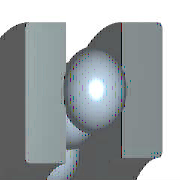
# Autodesk Inventor part: ISO 104 - 1 71 - 10 x 24 x 6
Saved by Autodesk Inventor 2023.3 (Build 273359000, 359)
## iProperties
Created: 2022-02-04
Part Number: ISO 104 - 1 71 - 10 x 24 x 6
Material: Steel, Mild
Description: Rolling bearing-Thrust bearing(Single Direction)
Document SubType Name: Modeling
Standard: ISO 104
Designer: Csábi-Kis Henrik
Standard Revision: Third edition 2002-02-01
Standards Organization: ISO
Language: en-US
Size Designation: 1 71 - 10 x 24 x 6
Categories: <MemberInstance><Categories><Category DisplayName="Shaft Parts" InternalName="7f7aeb1f-a693-4053-b835-cee3144e0d98" Mnemonic="SHFT"><Category DisplayName="Bearings" InternalName="242d30a3-7172-44e6-a363-b0a3d8f1b556" Mnemonic="BRNG"><CategoryParameter DisplayName="Width" InternalName="25fc5f6e-338b-4801-b5ed-8959743e396e" Mnemonic="wdth"/><CategoryParameter DisplayName="Size Designation" InternalName="2c4e891a-c8f4-49ed-a5c1-5131476c6feb" Mnemonic="sizedes"/><CategoryParameter DisplayName="Basic Dynamic Load Rating" InternalName="440972dd-7009-4861-bd45-69ffbb461423" Mnemonic="bdynlrat"/><CategoryParameter DisplayName="Shaft Diameter" InternalName="91302473-2833-4451-a660-c5d4a8d6a031" Mnemonic="shaftdia"/><CategoryParameter DisplayName="Touch Angle" InternalName="aa21a452-7974-4a55-b5cf-1c2972de2aea" Mnemonic="TouchAngle"/><CategoryParameter DisplayName="Outer Diameter" InternalName="d441686c-04bd-4681-b674-94fbc173ec23" Mnemonic="outdia"/><Category DisplayName="Ball Bearings" InternalName="9b553946-0899-4a5e-a403-c1d9295e77c1" Mnemonic="BALLBEAR"><CategoryParameter DisplayName="Radial Dynamic Load Factor when Fa/Fr &lt;= e" InternalName="051e59b3-bd55-4dad-8b07-38b5cb912881" Mnemonic="raddynfc1"/><CategoryParameter DisplayName="Basic Static Load Rating" InternalName="0f13fbbf-c511-4d43-b4c7-197b47424baf" Mnemonic="bstatlrat"/><CategoryParameter DisplayName="Exponent for Determining Life" InternalName="3029e2ef-9460-4be8-bdfd-dfe61437473d" Mnemonic="lifeexp"/><CategoryParameter DisplayName="Friction Factor" InternalName="3086b0f2-3d69-46ff-8a75-fe12e395bb47" Mnemonic="fricfct"/><CategoryParameter DisplayName="Min. Shaft Diameter" InternalName="4a5be9bc-ad86-4bf2-8167-102dad5d3e27" Mnemonic="minshaftdia"/><CategoryParameter DisplayName="Axial Dynamic Load Factor when Fa/Fr &gt; e" InternalName="4b6ff741-5956-4a40-80f5-34eb9259f88c" Mnemonic="axdynfc2"/><CategoryParameter DisplayName="Limiting Speed Lubrication Grease" InternalName="5237843b-2c8d-46d3-8227-f3e9dd85a12e" Mnemonic="lubgrsp"/><CategoryParameter DisplayName="Limiting Speed Oil" InternalName="60628548-8907-44dc-8e09-603d72f5766f" Mnemonic="oilspd"/><CategoryParameter DisplayName="Axial Static Load Factor" InternalName="74dbf5e2-8362-409a-802f-3c2235668d99" Mnemonic="axdynfc0"/><CategoryParameter DisplayName="Mass" InternalName="7b80f85c-da81-4dea-b8db-d7c689da91b2" Mnemonic="mass"/><CategoryParameter DisplayName="Radius" InternalName="83352640-dfae-4cba-bc9f-11ecbfb0001c" Mnemonic="rad"/><CategoryParameter DisplayName="Radial Static Load Factor" InternalName="83ce084d-c51e-4598-a871-e8e1e34b26ee" Mnemonic="raddynfc0"/><CategoryParameter DisplayName="Axial Dynamic Load Factor when Fa/Fr &lt;= e" InternalName="ae45a7db-08df-4411-99a8-2f035015bff9" Mnemonic="axdynfc1"/><CategoryParameter DisplayName="Max. Hub Step Diameter" InternalName="b5cf89e0-ca87-439c-b08c-a25e2999ab06" Mnemonic="maxhubdia"/><CategoryParameter DisplayName="Limiting Value for Factor Determination" InternalName="be0ce6fc-cad4-4218-b484-c34dd2571812" Mnemonic="limvalfac"/><CategoryParameter DisplayName="Radial Dynamic Load Factor when Fa/Fr &gt; e" InternalName="e513bdb7-139f-4b3c-af32-49e0ba1226b9" Mnemonic="raddynfc2"/><CategoryParameter DisplayName="Max. Step Fillet Radius" InternalName="f6ce6695-cf2c-4ec9-8d20-66671e0e35a4" Mnemonic="maxstprad"/><Category DisplayName="Thrust Ball Bearings" InternalName="fd9b3ea9-37cc-4212-9aeb-e74e3b8fad91" Mnemonic="BBTBB"/></Category></Category></Category><Category DisplayName="DataType" InternalName="23b78d0f-2648-40c6-8793-ca6db495c9e8" Mnemonic="DATATYPE"><CategoryParameter DisplayName="DisplayName" InternalName="05415f3d-3907-474b-a020-eb9d644f4cf3" Mnemonic="DISPLAYNAME"/><CategoryParameter DisplayName="Standard" InternalName="0c0a119c-1e12-4c84-803f-101930972f5e" Mnemonic="STANDARD"/><CategoryParameter DisplayName="Description" InternalName="13903e3d-64b1-4950-80da-f627842ea37f" Mnemonic="DESCRIPTION"/><CategoryParameter DisplayName="Designation" InternalName="2675968c-4ce5-49e0-a4f5-552d29089031" Mnemonic="DESIGNATION"/><CategoryParameter DisplayName="Default Row" InternalName="2af9ec52-faaa-4026-b378-f9fa4afca842" Mnemonic="DEFAULTROW"/><CategoryParameter DisplayName="Folder Name" InternalName="3f06958e-8713-4116-9be7-ed6184ecc97b" Mnemonic="FOLDERNAME"/><CategoryParameter DisplayName="Revision Guid" InternalName="45a75005-10b1-4dfc-8d6d-dfe629f0b93c" Mnemonic="REVISIONGUID"/><CategoryParameter DisplayName="FileName" InternalName="8b46a4cc-9585-4fed-90c3-899f57e09a73" Mnemonic="FILENAME"/><CategoryParameter DisplayName="StdsOrg" InternalName="8f5914e1-4693-403f-8ab5-d37768198c9d" Mnemonic="STDSORG"/><CategoryParameter DisplayName="Family Version" InternalName="914462f6-6e19-4b14-ba84-155b9680b1d0" Mnemonic="FAMILYREVISION"/><CategoryParameter DisplayName="Standard Revision" InternalName="91d5a463-65c2-4fde-b823-3b7fea5e8e17" Mnemonic="STANDARDREVISION"/><CategoryParameter DisplayName="Member Revision" InternalName="a65d44b9-392f-4f4f-857b-e4b3d54996fe" Mnemonic="MEMBERREVISION"/><CategoryParameter DisplayName="ClipFormat" InternalName="bc51e27b-3422-4e78-93ef-cec197ddf230" Mnemonic="CLIPFORMAT"/><CategoryParameter DisplayName="Manufacturer" InternalName="cd6c7a72-a28a-4e50-99a9-2c7f4e13e5ad" Mnemonic="MANUFACTURER"/><CategoryParameter DisplayName="InternalName" InternalName="cf1d0246-76d9-4b4a-8305-fa0409afb5c1" Mnemonic="INTERNALNAME"/><CategoryParameter DisplayName="IsMetric" InternalName="e2385c5b-1ea4-4823-96a8-8de651266ec3" Mnemonic="ISMETRIC"/><Category DisplayName="Part" InternalName="c0e0b642-3bcb-4cc8-9e80-f96d35c4afa4" Mnemonic="PART"><CategoryParameter DisplayName="Part Number" InternalName="016b6077-bfbe-49bd-92c9-d8d59c39c941" Mnemonic="PARTNUMBER"/><CategoryParameter DisplayName="Stock Number" InternalName="4dba7c1c-e26c-444e-836c-b08b433409a8" Mnemonic="STOCKNUMBER"/><CategoryParameter DisplayName="Material Key" InternalName="5c9a8adb-dd2b-4535-b97f-0a94a95fe41f" Mnemonic="MATERIALKEY"/><CategoryParameter DisplayName="Material" InternalName="818a152a-d3c3-49ca-80ee-df7d91421b8e" Mnemonic="MATERIAL"/></Category></Category><Category DisplayName="LegacyMap" InternalName="cd87c42b-3e48-431e-b5c0-1cbeb14dfe77" Mnemonic="LEGACYMAP"><CategoryParameter DisplayName="unique DA member ID" InternalName="0918ad47-427f-4fed-ae26-24c81c58f590" Mnemonic="DACOOKIE"/><CategoryParameter DisplayName="Merge11 ID" InternalName="0ee8fb18-e2ed-4f39-96f6-1f4b5f50aa71" Mnemonic="MERGE11"/><CategoryParameter DisplayName="unique CC member ID" InternalName="5193edd4-b2b0-4ab4-9d54-de900eee34e0" Mnemonic="CCCOOKIE"/><CategoryParameter DisplayName="Split ID" InternalName="72b5c83c-be7f-45c4-ae51-9160ea6deb26" Mnemonic="SPLIT"/><CategoryParameter DisplayName="MemberID" InternalName="8e5e0294-fc51-4c8f-b3d7-003dc5ed94f6" Mnemonic="MEMBERID"/><CategoryParameter DisplayName="CatalogName" InternalName="d99d1e27-aa94-4de2-af4c-c348882a6f4f" Mnemonic="CATALOGNAME"/><CategoryParameter DisplayName="FamilyNumber" InternalName="e705e1f4-09cb-413e-91f9-551b4188271e" Mnemonic="FAMILYNUMBER"/></Category></Categories><FamilyTemplate Id="ba0018"><FamilyTemplateParameters><FamilyTemplateParameter ObjectType="kUserParameterObject" ValueType="xs:double" Id="1" ObjectReferenceKey="WR"/><FamilyTemplateParameter ObjectType="kUserParameterObject" ValueType="xs:double" Id="2" ObjectReferenceKey="BC"/><FamilyTemplateParameter ObjectType="kUserParameterObject" ValueType="xs:double" Id="3" ObjectReferenceKey="KRS"/><FamilyTemplateParameter ObjectType="kUserParameterObject" ValueType="xs:double" Id="4" ObjectReferenceKey="WD"/><FamilyTemplateParameter ObjectType="kUserParameterObject" ValueType="xs:double" Id="5" ObjectReferenceKey="KAD1"/><FamilyTemplateParameter ObjectType="kUserParameterObject" ValueType="xs:double" Id="6" ObjectReferenceKey="KB"/><FamilyTemplateParameter ObjectType="kUserParameterObject" ValueType="xs:double" Id="7" ObjectReferenceKey="BBA"/><FamilyTemplateParameter ObjectType="kUserParameterObject" ValueType="xs:double" Id="8" ObjectReferenceKey="BC0"/><FamilyTemplateParameter ObjectType="kUserParameterObject" ValueType="xs:double" Id="9" ObjectReferenceKey="BD"/><FamilyTemplateParameter ObjectType="kUserParameterObject" ValueType="xs:double" Id="10" ObjectReferenceKey="BR"/><FamilyTemplateParameter ObjectType="kUserParameterObject" ValueType="xs:double" Id="11" ObjectReferenceKey="KID1"/><FamilyTemplateParameter ObjectType="kUserParameterObject" ValueType="xs:double" Id="12" ObjectReferenceKey="BI"/><FamilyTemplateParameter ObjectType="kPropertyObject" ValueType="xs:string" Id="100" ObjectReferenceKey="{32853F0F-3444-11d1-9E93-0060B03C1CA6}" SubObjectId="52"/><FamilyTemplateParameter ObjectType="kPropertyObject" ValueType="xs:string" Id="105" ObjectReferenceKey="{32853F0F-3444-11d1-9E93-0060B03C1CA6}" SubObjectId="5"/><FamilyTemplateParameter ObjectType="kPartComponentDefinitionObject" ValueType="xs:string" Id="110" SubObjectId="Material"/></FamilyTemplateParameters></FamilyTemplate><CategoryParameterMap><ParamToTemplateMap><ParamToTemplate CategoryParameter="//CategoryParameter[@InternalName='05415f3d-3907-474b-a020-eb9d644f4cf3']" ConstantValue="ISO 104 (Single Direction)"/><ParamToTemplate CategoryParameter="//CategoryParameter[@InternalName='cf1d0246-76d9-4b4a-8305-fa0409afb5c1']" ConstantValue="14b0c8a4-116f-4d89-bad3-372984a9f60c"/><ParamToTemplate CategoryParameter="//CategoryParameter[@InternalName='3f06958e-8713-4116-9be7-ed6184ecc97b']" ConstantValue="ISO 104"/><ParamToTemplate CategoryParameter="//CategoryParameter[@InternalName='914462f6-6e19-4b14-ba84-155b9680b1d0']" ConstantValue="10"/><ParamToTemplate CategoryParameter="//CategoryParameter[@InternalName='bc51e27b-3422-4e78-93ef-cec197ddf230']" ConstantValue="CF_INVENTOR.STDPARTS"/><ParamToTemplate CategoryParameter="//CategoryParameter[@InternalName='e2385c5b-1ea4-4823-96a8-8de651266ec3']" ConstantValue="true"/><ParamToTemplate CategoryParameter="//CategoryParameter[@InternalName='13903e3d-64b1-4950-80da-f627842ea37f']" ConstantValue="Rolling bearing-Thrust bearing(Single Direction)"/><ParamToTemplate CategoryParameter="//CategoryParameter[@InternalName='8f5914e1-4693-403f-8ab5-d37768198c9d']" ConstantValue="ISO"/><ParamToTemplate CategoryParameter="//CategoryParameter[@InternalName='0c0a119c-1e12-4c84-803f-101930972f5e']" ConstantValue="ISO 104"/><ParamToTemplate CategoryParameter="//CategoryParameter[@InternalName='cd6c7a72-a28a-4e50-99a9-2c7f4e13e5ad']" TemplateParameter="104"/><ParamToTemplate CategoryParameter="//CategoryParameter[@InternalName='91d5a463-65c2-4fde-b823-3b7fea5e8e17']" ConstantValue="Third edition 2002-02-01"/><ParamToTemplate CategoryParameter="//CategoryParameter[@InternalName='45a75005-10b1-4dfc-8d6d-dfe629f0b93c']" ConstantValue="254451d5-769d-4a13-b570-04789f9de70c"/><ParamToTemplate CategoryParameter="//CategoryParameter[@InternalName='2af9ec52-faaa-4026-b378-f9fa4afca842']" ConstantValue="10"/><ParamToTemplate CategoryParameter="//CategoryParameter[@InternalName='d99d1e27-aa94-4de2-af4c-c348882a6f4f']" ConstantValue="ISO"/><ParamToTemplate CategoryParameter="//CategoryParameter[@InternalName='e705e1f4-09cb-413e-91f9-551b4188271e']" ConstantValue="112"/><ParamToTemplate CategoryParameter="//CategoryParameter[@InternalName='8b46a4cc-9585-4fed-90c3-899f57e09a73']" ConstantValue="ISO 104 - 1 71 - 10 x 24 x 6"/><ParamToTemplate CategoryParameter="//CategoryParameter[@InternalName='a65d44b9-392f-4f4f-857b-e4b3d54996fe']" ConstantValue="9b549998-5bd1-48f5-9ed4-53cb02577c6e"/><ParamToTemplate CategoryParameter="//CategoryParameter[@InternalName='2c4e891a-c8f4-49ed-a5c1-5131476c6feb']" ConstantValue="1 71 - 10 x 24 x 6"/><ParamToTemplate CategoryParameter="//CategoryParameter[@InternalName='8e5e0294-fc51-4c8f-b3d7-003dc5ed94f6']" ConstantValue="210"/><ParamToTemplate CategoryParameter="//CategoryParameter[@InternalName='aa21a452-7974-4a55-b5cf-1c2972de2aea']" TemplateParameter="7"/><ParamToTemplate CategoryParameter="//CategoryParameter[@InternalName='440972dd-7009-4861-bd45-69ffbb461423']" TemplateParameter="2"/><ParamToTemplate CategoryParameter="//CategoryParameter[@InternalName='0f13fbbf-c511-4d43-b4c7-197b47424baf']" TemplateParameter="8"/><ParamToTemplate CategoryParameter="//CategoryParameter[@InternalName='d441686c-04bd-4681-b674-94fbc173ec23']" TemplateParameter="9"/><ParamToTemplate CategoryParameter="//CategoryParameter[@InternalName='2675968c-4ce5-49e0-a4f5-552d29089031']" TemplateParameter="100"/><ParamToTemplate CategoryParameter="//CategoryParameter[@InternalName='25fc5f6e-338b-4801-b5ed-8959743e396e']" TemplateParameter="6"/><ParamToTemplate CategoryParameter="//CategoryParameter[@InternalName='83352640-dfae-4cba-bc9f-11ecbfb0001c']" TemplateParameter="3"/><ParamToTemplate CategoryParameter="//CategoryParameter[@InternalName='818a152a-d3c3-49ca-80ee-df7d91421b8e']" TemplateParameter="110"/><ParamToTemplate CategoryParameter="//CategoryParameter[@InternalName='016b6077-bfbe-49bd-92c9-d8d59c39c941']" TemplateParameter="105"/><ParamToTemplate CategoryParameter="//CategoryParameter[@InternalName='91302473-2833-4451-a660-c5d4a8d6a031']" TemplateParameter="4"/></ParamToTemplateMap></CategoryParameterMap></MemberInstance>
Density: 7.85 g/cm^3
Appearance: Semi-Polished
IsCustomPart: 0
Author: Csábi-Kis Henrik
Autodesk Inventor part; units mm, degrees
note: some values were not read from the file. Left out: dimensions or parameters whose unit could not be read.
ref_plane "YZ Plane" through (0, 0, 0) normal (1, 0, 0) x (0, 1, 0)
ref_plane "XZ Plane" through (0, 0, 0) normal (0, 1, 0) x (-1, 0, 0)
ref_plane "XY Plane" through (0, 0, 0) normal (0, 0, 1) x (1, 0, 0)
sketch "Sketch" plane through (0, 0, 0) normal (0, 0, 1) x (1, 0, 0)
  line L0 (3, 7.18) -> (3, 9.82) construction
  line L1 (4.32, 8.5) -> (1.68, 8.5)
  circle A0 centre (3, 8.5) radius 1.32
  line L2 (1.8, 9.049909) -> (1.8, 12)
  line L3 (1.8, 12) -> (0, 12)
  line L4 (1.8, 5) -> (0, 5)
  line L5 (4.2, 9.049909) -> (4.2, 12)
  line L6 (4.2, 12) -> (6, 12)
  line L7 (6, 12) -> (6, 5)
  line L8 (6, 5) -> (4.2, 5)
  line L9 (4.2, 5) -> (4.2, 7.950091)
  line L10 (1.8, 7.950091) -> (1.8, 5)
  line L11 (-0.8, 0) -> (4.8, 0)
  line L12 (0, -0.107) -> (0, 2.357)
  dimension "d3" = 2.64
  dimension "d8" = 10
  dimension "d11" = 10
  dimension "d12" = 17
  dimension "d13" = 24
  dimension "d14" = 24
  dimension "d15" = 3
  dimension "d16" = 6
  dimension "d18" = 1.8
  constraints: 22 end point, 5 perpendicular, 3 collinear, 3 parallel, 2 midpoint, 2 point on line, 10 other
  measures "d8" diameter of L4 L11
  measures "d11" diameter of L8 L11
  measures "d12" diameter of point (3, 8.5) L11
  measures "d13" diameter of L3 L11
  measures "d14" diameter of L6 L11
  measures "d15" distance from line of L12 point (3, 8.5)
  measures "d16" distance between parallel lines of L12 L7
  measures "d18" distance between parallel lines of L12 L10
sketch "Sketch outline for Body" plane through (0, 0, 0) normal (0, 0, 1) x (1, 0, 0)
  arc A0 (1.8, 7.950091) -> (1.8, 9.049909) centre (3, 8.5) cw
  line L0 (1.8, 9.049909) -> (1.8, 12)
  line L1 (1.8, 12) -> (0, 12)
  line L2 (0, 12) -> (0, 5)
  line L3 (0, 5) -> (1.8, 5)
  line L4 (1.8, 5) -> (1.8, 7.950091)
  arc A1 (4.2, 9.049909) -> (4.2, 7.950091) centre (3, 8.5) cw
  line L5 (4.2, 7.950091) -> (4.2, 5)
  line L6 (4.2, 5) -> (6, 5)
  line L7 (6, 5) -> (6, 12)
  line L8 (6, 12) -> (4.2, 12)
  line L9 (4.2, 12) -> (4.2, 9.049909)
revolve "Body" add sketch "Sketch outline for Body" angle 360 about axis through (-10, 0, 0) along (1, 0, 0)
fillet "Fillet1" radius 0.3 2 edges at (0, -12, 0) (6, -12, 0)
fillet "Fillet2" radius 0.3 2 edges at (0, -5, 0) (6, -5, 0)
sketch "Sketch outline for Ball" plane through (0, 0, 0) normal (0, 0, 1) x (1, 0, 0)
  arc A0 (1.8, 7.950091) -> (3, 7.18) centre (3, 8.5) ccw
  arc A1 (1.68, 8.5) -> (1.8, 7.950091) centre (3, 8.5) ccw
  line L0 (4.32, 8.5) -> (1.68, 8.5)
  arc A2 (4.2, 7.950091) -> (4.32, 8.5) centre (3, 8.5) ccw
  arc A3 (3, 7.18) -> (4.2, 7.950091) centre (3, 8.5) ccw
revolve "Ball" add sketch "Sketch outline for Ball" angle 360 about axis through (4.32, 8.5, 0) along (-1, 0, 0)
pattern_circular "Balls" count 10 over 360 about axis through (-10, 0, 0) along (1, 0, 0) of "Ball"
equation "\"d3\" = 0.44 * KB"
equation "\"d8\" = WD"
equation "\"d11\" = KAD1"
equation "\"d12\" = 0.5 * KAD1 + 0.5 * KID1"
equation "\"d13\" = KID1"
equation "\"d14\" = BD"
equation "\"d15\" = 0.5 * KB"
equation "\"d16\" = KB"
equation "\"d18\" = 0.3 * KB"
equation "\"d4\" = KRS"
equation "\"d5\" = KRS"
equation "\"WD\" = 10"
equation "\"KAD1\" = 10"
equation "\"KID1\" = 24"
equation "\"BD\" = 24"
equation "\"KB\" = 6"
equation "\"KRS\" = 0.3"
equation "\"d0\" = 0.2 * KB"
equation "\"WR\" = 0.5 * WD"
equation "\"BBA\" = 90deg"
equation "\"BR\" = 0.5 * BD"
body "Solid1"
